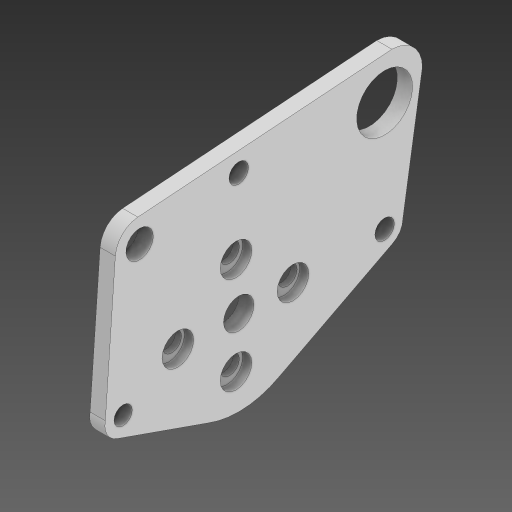
# Autodesk Inventor part: drib_lef
Saved by Autodesk Inventor 2023 (Build 270158000, 158)
## iProperties
Created: 2025-05-23
Part Number: drib_lef
Material: Типовые
Document SubType Name: Sheet Metal
Designer: daa
Density: 1 g/cm^3
Appearance: По умолчанию
Sheet Metal Rule: По умолчанию
Author: daa
Autodesk Inventor part; units mm, degrees
ref_plane "YZ Plane" through (0, 0, 0) normal (1, 0, 0) x (0, 1, 0)
ref_plane "XZ Plane" through (0, 0, 0) normal (0, 1, 0) x (-1, 0, 0)
ref_plane "XY Plane" through (0, 0, 0) normal (0, 0, 1) x (1, 0, 0)
sketch "Эскиз1" plane through (0, 0, 0) normal (1, 0, 0) x (0, 1, 0)
  circle A0 centre (25.7199, 46.7921) radius 2.25
  circle A1 centre (25.6987, 6.5017) radius 4.6
  circle A2 centre (7.6987, 6.5017) radius 1.6
  arc A3 (27.6873, 0.2956) -> (32.7199, 5.2955) centre (27.7199, 5.2955) ccw
  circle A4 centre (7.6843, 30.491) radius 14
  arc A5 (14.2267, 42.8683) -> (-1.4853, 19.9118) centre (7.6843, 30.491) ccw
  circle A6 centre (27.6987, 30.491) radius 1.6
  line L0 (7.6843, 30.491) -> (25.6987, 6.5017)
  line L1 (-6.3157, 30.491) -> (21.6843, 30.491)
  line L2 (7.6843, 16.491) -> (7.6843, 44.491)
  circle A7 centre (7.6843, 30.491) radius 2.5
  circle A8 centre (-0.3157, 30.491) radius 1.6
  circle A9 centre (15.6843, 30.491) radius 1.6
  circle A10 centre (7.6843, 20.991) radius 1.6
  circle A11 centre (7.6843, 39.991) radius 1.6
  circle A12 centre (2.6987, 49.5017) radius 1.5
  circle A13 centre (7.6987, 6.5017) radius 3
  line L3 (7.6987, 3.5017) -> (27.6873, 0.2956)
  circle A14 centre (2.6987, 49.5017) radius 3
  line L4 (-3.2958, 40.9198) -> (-5.3755, 35.5348)
  line L5 (-0.0999, 50.5825) -> (-5.3755, 35.5348)
  line L6 (-1.3769, 17.8835) -> (-4.5981, 23.7723)
  line L7 (-4.5981, 23.7723) -> (5.0667, 5.062)
  circle A15 centre (25.7199, 46.7921) radius 4
  line L8 (2.4504, 52.4914) -> (23, 51)
  line L9 (2.4504, 52.4914) -> (26.0094, 50.7816)
  line L10 (32.7199, 5.2955) -> (29.7095, 47.0795)
  point P0 (0, 0)
  point P1 (-2.3427, 0)
  point P2 (7.6843, 30.491)
  point P3 (7.6843, 30.491)
  point P4 (-4.5981, 23.7723)
  point P5 (-3.3371, 41.4181)
  point P6 (-5.3755, 35.5348)
  point P7 (5.0013, 5.1886)
  point P8 (-0.1621, 50.405)
  point P9 (3.376, 52.4242)
  dimension "d9" = 4.5
  dimension "d86" = 9.2
  dimension "d87" = 3.2
  dimension "d92" = 5
  dimension "d132" = 28
  dimension "d145" = 3.2
  dimension "d191" = 30
  dimension "d194" = 5
  dimension "d195" = 3.2
  dimension "d196" = 3.2
  dimension "d197" = 3.2
  dimension "d198" = 3.2
  dimension "d199" = 8
  dimension "d200" = 8
  dimension "d201" = 9.5
  dimension "d202" = 9.5
  dimension "d227" = 3
  dimension "d234" = 6
  dimension "d235" = 6
  dimension "d242" = 8
  constraints: 22 end point, 18 point on circle, 16 centre point, 7 coincident, 4 point on line, 3 tangent, 2 concentric, 2 midpoint, 1 horizontal, 1 perpendicular
  measures "d9" diameter of A0
  measures "d86" diameter of A1
  measures "d87" diameter of A2
  measures "d92" radius of A3
  measures "d132" diameter of A4
  measures "d145" diameter of A6
  measures "d191" distance of L0.start L0.end
  measures "d194" diameter of A7
  measures "d195" diameter of A8
  measures "d196" diameter of A9
  measures "d197" diameter of A10
  measures "d198" diameter of A11
  measures "d199" distance of A8.centre point (7.684, 30.491)
  measures "d200" distance of point (7.684, 30.491) A9.centre
  measures "d201" distance of A4.centre A10.centre
  measures "d202" distance of A4.centre A11.centre
  measures "d227" diameter of A12
  measures "d234" diameter of A13
  measures "d235" diameter of A14
  measures "d242" diameter of A15
extrude "Выдавливание1" add sketch "Эскиз1" along normal blind 2.5 contours L3 A13 L7 A4 L5 A14 L8 L9 A15 L10 A3 | A13 | A15 | A4 L1 A8 A7 L2 A10 | A4 L2 A11 A7 L1 A8 | L8 A14 | L2 A10 A7 L0 A4 | A4 L1 A9 A7 L2 A11 | L0 A7 L1 A9 A4
sketch "Эскиз8" plane through (2.5, 0, 0) normal (1, 0, 0) x (0, 0, -1)
  circle A0 centre (-40.5072, 7.6405) radius 1.6
  circle A1 centre (-40.5072, 7.6405) radius 2.6
  circle A2 centre (-30.9442, -0.3839) radius 1.6
  circle A3 centre (-30.9442, -0.3839) radius 2.6
  circle A4 centre (-21.5765, 7.6255) radius 1.6
  circle A5 centre (-21.5765, 7.6255) radius 2.6
  circle A6 centre (-30.9442, 15.6084) radius 1.6
  circle A7 centre (-30.9442, 15.6084) radius 2.6
  point P0 (0, 0)
  dimension "d205" = 3.2
  dimension "d206" = 5.2
  dimension "d207" = 3.2
  dimension "d208" = 5.2
  dimension "d210" = 3.2
  dimension "d211" = 5.2
  dimension "d216" = 3.2
  dimension "d217" = 5.2
  constraints: 8 centre point, 4 coincident
  measures "d205" diameter of A0
  measures "d206" diameter of A1
  measures "d207" diameter of A2
  measures "d208" diameter of A3
  measures "d210" diameter of A4
  measures "d211" diameter of A5
  measures "d216" diameter of A6
  measures "d217" diameter of A7
extrude "Выдавливание9" cut sketch "Эскиз8" against normal blind 1.5 contours A0 | A1 | A2 | A3 | A4 | A5 | A6 | A7
equation "\"Радиус_гибки\" = Толщина"
equation "\"Ширина_просечки\" = Толщина"
equation "\"Глубина_просечки\" = 0.5 * Толщина"
equation "\"Размер_просечки\" = 4 * Толщина"
equation "\"Мин_остаток\" = 2 * Толщина"
equation "\"Радиус_перехода\" = Радиус_гибки"
equation "\"Радиус_Якоби\" = Радиус_гибки"
equation "\"Размер_зазора\" = Толщина"
equation "\"Толщина\" = 3.048"
